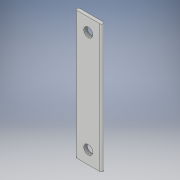
# Autodesk Inventor part: Part I
Saved by Autodesk Inventor 2018 (Build 220112000, 112)
## iProperties
Created: 2018-10-04
Part Number: Part I
Material: Generic
Document SubType Name: Modeling
Designer: Jayden
Density: 1 g/cm^3
Appearance: Default
Author: Jayden
Autodesk Inventor part; units mm, degrees
ref_plane "YZ Plane" through (0, 0, 0) normal (1, 0, 0) x (0, 1, 0)
ref_plane "XZ Plane" through (0, 0, 0) normal (0, 1, 0) x (-1, 0, 0)
ref_plane "XY Plane" through (0, 0, 0) normal (0, 0, 1) x (1, 0, 0)
sketch "Sketch1" plane through (0, 0, 0) normal (0, 0, 1) x (1, 0, 0)
  circle A0 centre (0, 24.5) radius 2.1828
  circle A1 centre (0, -24.5) radius 2.1828
  line L0 (6.35, -30.85) -> (-6.35, -30.85)
  line L1 (-6.35, -30.85) -> (-6.35, 30.85)
  line L2 (-6.35, 30.85) -> (6.35, 30.85)
  line L3 (6.35, 30.85) -> (6.35, -30.85)
  line L4 (6.35, -30.85) -> (-6.35, 30.85) construction
  line L5 (-6.35, -30.85) -> (6.35, 30.85) construction
  point P0 (0, 0)
  dimension "d0" = 4.3656
  dimension "d1" = 4.3656
  dimension "d2" = 49
  dimension "d3" = 24.5
  dimension "d4" = 24.5
  dimension "d5" = 12.7
  dimension "d6" = 6.35
  dimension "d7" = 6.35
  constraints: 12 end point, 2 centre point, 2 midpoint, 2 parallel, 1 horizontal, 1 perpendicular
  measures "d0" diameter of A0
  measures "d1" diameter of A1
  measures "d2" distance of A0.centre A1.centre
  measures "d3" distance of point (0, 0) A0.centre
  measures "d4" distance of point (0, 0) A1.centre
  measures "d5" distance of L1.end L2.end
  measures "d6" distance from line of L2 A0.centre
  measures "d7" distance from line of L0 A1.centre
extrude "Extrusion1" add sketch "Sketch1" along normal blind 1.5875
fillet "Fillet1" radius 0.7937 4 edges at (6.35, 0, 1.5875) (6.35, 0, 0) (-6.35, 0, 0) (-6.35, 0, 1.5875)
body "Solid1"
